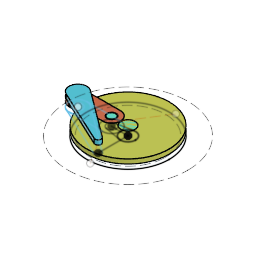
Test (Autodesk Fusion 360 design; units mm, degrees)
Autodesk Fusion 360 part; units mm, degrees
note: some values were not read from the file. Chosen so that the rebuilt part matches the saved one: which face or edge a step refers to. Set by a fixed rule: which sketch regions a step uses.
sketch "Sketch1" plane through (0, 0, 0) normal (0, 0, 1) x (1, 0, 0)
  circle A0 centre (0, 0) radius 27.5
  circle A1 centre (0, 0) radius 5
  circle A2 centre (-11, 0) radius 6
  circle A3 centre (-33.5, 0) radius 6
  line L0 (-33.5, 6) -> (-11, 6)
  circle A4 centre (0, 0) radius 25 construction
  circle A5 centre (0, 0) radius 40 construction
  line L1 (0, 0) -> (-11, 0)
  line L2 (-33.5, -6) -> (-11, -6)
  circle A6 centre (-33.5, 0) radius 3
  circle A7 centre (-11, 0) radius 3
  line L3 (-11, -6) -> (3.3584, -28.6291) construction
  line L4 (-11, 6) -> (3.3584, 28.6291) construction
  line L5 (0, 0) -> (0, -20)
  circle A8 centre (0, -20) radius 1
  circle A9 centre (0, -20) radius 2
  line L6 (-0.8438, -21.8133) -> (-36.0313, -5.4399)
  circle A10 centre (0, 0) radius 5
  line L7 (0, -5.0848) -> (-11.5455, -2.95)
  line L8 (-11.5455, 2.95) -> (-0.9091, 4.9167)
  line L9 (1.1959, -18.3969) -> (-31.5086, 6)
  dimension "d1" = 55
  dimension "d2" = 10
  dimension "d4" = 12
  dimension "d8" = 12
  dimension "d10" = 50
  dimension "d11" = 80
  dimension "d12" = 6
  dimension "d13" = 6
  dimension "d16" = 26.8
  dimension "d17" = 26.8
  dimension "d18" = 20
  dimension "d19" = 2
  dimension "d20" = 4
  dimension "d21" = 10
  constraint coincident A0.centre A1.centre
  constraint concentric A0 A1
  constraint tangent A1 A2
  constraint tangent A0 A3
  constraint concentric A1 A4
  constraint coincident A2.centre L1.end
  constraint horizontal L1
  constraint tangent A2 L0
  constraint tangent A3 L0
  constraint coincident A3 L0.start
  constraint coincident A2 L0.end
  constraint tangent A3 L2
  constraint coincident A2 L2.end
  constraint coincident A3 L2.start
  constraint tangent A2 L2
  constraint concentric A3 A6
  constraint tangent A3 L6
  constraint perpendicular L1 L5
  constraint coincident L5.end A8.centre
  constraint concentric A8 A9
  constraint tangent A9 L6
  constraint coincident A3 L6.end
  constraint coincident A9 L6.start
  constraint concentric A0 A10
  constraint tangent A7 L8
  constraint tangent A7 L7
  constraint tangent A10 L7
  constraint tangent A10 L8
  constraint coincident A7 L7.end
  constraint coincident A7 L8.start
  constraint coincident A10 L8.end
  constraint coincident L5 L7.start
  constraint tangent A3 L9
  constraint tangent A9 L9
  constraint coincident L0 L9.end
  constraint coincident A9 L9.start
  measures "d1" diameter of A0
  measures "d2" diameter of A1
  measures "d4" diameter of A2
  measures "d8" diameter of A3
  measures "d10" diameter of A4
  measures "d11" diameter of A5
  measures "d12" diameter of A6
  measures "d13" diameter of A7
  measures "d16" distance of L2.end L3.end
  measures "d17" distance of L0.end L4.end
  measures "d18" distance of A0.centre L5.end
  measures "d19" diameter of A8
  measures "d20" diameter of A9
  measures "d21" diameter of A10
extrude "Extrude1" add sketch "Sketch1" along normal blind 3 contours A1 A2 A10 L8 | A2 L1 A7 L8 | A2 L1 A7 L7 | A1 A2 A10 L7 | A1 L1 L5 A10 | A1 L1 L5 A10 | A7 makes body 1 in component "Base"
extrude "Extrude2" add sketch "Sketch1" along normal blind 6 contours A1 L1 L5 A10 | A1 L1 L5 A10 bodies 1 in component "Base"
extrude "Extrude1'" add sketch "Sketch1" along normal blind 3 from surface at 3 separate body contours A0 A1 A2 L0 L5 A9 L6 A10 L8 L9 | A0 L2 L5 A9 L6 L9 | A9 | A2 L2 L5 L7 L9 | A1 A2 A10 L8 | A1 A2 A10 L7 | A1 L1 L5 A10 | A1 L1 L5 A10 | A1 L5 A10 L7 makes body 2 in component "Centre"
extrude "Extrude1''" add sketch "Sketch1" along normal blind 3 from surface at 3 separate body contours A0 A2 L0 L2 L9 | A0 L0 L9 | A0 L2 L9 | A0 A3 L9 | A3 L0 L9 | A2 A7 L7 L8 | A0 A3 L2 | A3 | A2 L1 A7 L8 | A2 L1 A7 L7 makes body 3 in component "OuterArm"
extrude "Extrude1'''" add sketch "Sketch1" along normal blind 3 from surface at 6 separate body contours A0 A3 L2 L6 | A0 L2 L5 A9 L6 L9 | A0 L2 L9 | A0 A3 L9 | A0 A3 L2 | A9 | A3 | L5 A9 L9 | A6 | A8 makes body 4 in component "InnerArm"
extrude "Extrude2'" add sketch "Sketch1" along normal blind 3 from surface at 3 contours A6 | A8 bodies 4 in component "InnerArm"
extrude "Extrude3" add sketch "Sketch1" along normal blind 6 contours A7 bodies 1 in component "Base"
move_face "OffsetFaces1" offset -0.3 1 faces at (-30.5037, -0.1495, 5) on bodies 4 in component "InnerArm"
move_face "OffsetFaces2" offset -0.3 1 faces at (0.9988, -19.9502, 4) on bodies 4 in component "InnerArm"
move_face "OffsetFaces1'" offset -0.3 4 faces at (-11.873, -2.8702, 3) (-8, 3.6056, 2) (-4.4545, -4.2611, 1) (-0.0612, -4.9996, 4) on bodies 1 in component "Base"
component "Base" placed x (1, 0, 0) y (0, 1, 0) z (0, 0, 1) at (0, 0, 0)
component "Centre" placed x (1, 0, 0) y (0, 1, 0) z (0, 0, 1) at (0, 0, 0)
component "OuterArm" placed x (1, 0, 0) y (0, 1, 0) z (0, 0, 1) at (0, 0, 0)
component "InnerArm" placed x (1, 0, 0) y (0, 1, 0) z (0, 0, 1) at (0, 0, 0)
